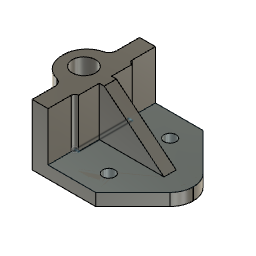
A3 v1 (Autodesk Fusion 360 design; units mm, degrees)
Autodesk Fusion 360 part; units mm, degrees
sketch "bottom" plane through (0, 0, 0) normal (0, 0, 1) x (1, 0, 0)
  line L0 (44, -44) -> (-44, -44)
  line L1 (-44, -44) -> (-44, 44)
  line L2 (-44, 44) -> (44, 44)
  line L3 (44, 44) -> (44, -44)
  line L4 (44, -44) -> (-44, 44) construction
  line L5 (-44, -44) -> (44, 44) construction
  dimension "d1" = 88
  dimension "d2" = 88
  constraint horizontal L0
  constraint perpendicular L0 L1
  constraint parallel L0 L2
  constraint parallel L1 L3
  constraint coincident L4 origin
  constraint coincident L5 origin
  measures "d1" distance of L1.end L2.end
  measures "d2" distance of L0.end L1.end
extrude "Extrude1" add sketch "bottom" along normal blind 10
sketch "Sketch2" plane through (0, 0, 10) normal (0, 0, 1) x (-1, 0, 0)
  line L0 (-44, -44) -> (44, -44)
  line L1 (44, -44) -> (44, 44)
  line L2 (44, 44) -> (-44, 44)
  line L3 (-44, 44) -> (-44, -44)
  line L4 (-44, 0) -> (-25, 0)
  circle A0 centre (-25, 0) radius 19
  constraint midpoint L3 L4.start
  constraint perpendicular L3 L4
  constraint coincident L4.end A0.centre
  constraint coincident L4.start A0
chamfer "Chamfer1" distance 36 angle 45 2 edges at (44, -44, 5) (44, 44, 5)
fillet "Fillet1" radius 19 2 edges at (44, -8, 5) (44, 8, 5)
sketch "Sketch3" plane through (0, 0, 10) normal (0, 0, 1) x (-1, 0, 0)
  line L0 (44, 44) -> (31, 44)
  line L1 (31, 44) -> (31, -44)
  line L2 (31, -44) -> (44, -44)
  line L3 (44, -44) -> (44, 44)
  constraint horizontal L0
  constraint vertical L1
  constraint horizontal L2
  constraint vertical L3
extrude "Extrude2" add sketch "Sketch3" along normal blind 40
sketch "Sketch4" plane through (0, 0, 10) normal (0, 0, 1) x (-1, 0, 0)
  line L0 (31, -44) -> (31, 44)
  line L1 (31, 44) -> (-8, 44)
  line L2 (-8, 44) -> (-38.435, 13.565)
  arc A0 (-38.435, 13.565) -> (-44, 0.1299) centre (-25, 0.1299) ccw
  line L3 (-44, 0.1299) -> (-44, -0.1299)
  arc A1 (-44, -0.1299) -> (-38.435, -13.565) centre (-25, -0.1299) ccw
  line L4 (-38.435, -13.565) -> (-8, -44)
  line L5 (-8, -44) -> (31, -44)
  line L6 (28, -22) -> (31, -22)
  line L7 (31, -22) -> (31, 22)
  line L8 (31, 22) -> (28, 22)
  line L9 (28, 22) -> (28, -22)
  dimension "d12" = 3
  constraint horizontal L6
  constraint vertical L7
  constraint horizontal L8
  constraint vertical L9
  constraint coincident L0 L7.end
  measures "d12" distance of L6.start L6.end
extrude "Extrude3" add sketch "Sketch4" along normal blind 40 contours L0 L6 L7 L8 L9
fillet "Fillet2" radius 3 1 edges at (-31, -22, 30)
fillet "Fillet3" radius 3 1 edges at (-31, 22, 30)
sketch "Sketch6" plane through (0, 0, 0) normal (0, 1, 0) x (1, 0, 0)
  line L0 (-28, -50) -> (-24, -50)
  line L1 (-24, -50) -> (-24, -10)
  line L2 (-24, -10) -> (-28, -10)
  line L3 (-28, -10) -> (-28, -50)
  dimension "d19" = 40
  constraint horizontal L0
  constraint vertical L1
  constraint horizontal L2
  constraint vertical L3
  measures "d19" distance of L0.end L1.end
extrude "Extrude4" add sketch "Sketch6" along normal mid plane 10
sketch "triangle" plane through (0, -5, 0) normal (0, -1, 0) x (1, 0, 0)
  line L0 (-28, 50) -> (-28, 10)
  line L1 (-28, 10) -> (-24, 10)
  line L2 (-24, 10) -> (-24, 50)
  line L3 (-24, 50) -> (-28, 50)
  line L4 (-24, 50) -> (-24, 10)
  line L5 (-24, 10) -> (25, 10)
  line L6 (25, 10) -> (-24, 50)
  line L7 (44, 10) -> (25, 10)
  dimension "d26" = 19
  dimension "d28" = 49
  constraint coincident L2.end L3.start
  constraint coincident L1.end L2.start
  constraint perpendicular L4 L5
  measures "d26" distance of L5.end L7.start
  measures "d28" distance of L1.end L5.end
extrude "Extrude5" add sketch "triangle" against normal blind 10 contours L2 L4 L5 L6
sketch "the back" plane through (-44, 0, 0) normal (-1, 0, 0) x (0, -1, 0)
  line L0 (-44, 0) -> (44, 0)
  line L1 (44, 0) -> (44, 50)
  line L2 (44, 50) -> (-44, 50)
  line L3 (-44, 50) -> (-44, 0)
  line L4 (-19, 50) -> (19, 50)
  line L5 (19, 50) -> (19, 0)
  line L6 (19, 0) -> (-19, 0)
  line L7 (-19, 0) -> (-19, 50)
  constraint coincident L2 L4.start
  constraint horizontal L4
  constraint vertical L5
  constraint horizontal L6
  constraint vertical L7
  constraint coincident L0 L5.end
extrude "Extrude6" add sketch "the back" along normal blind 19 contours L0 L2 L4 L5 L6 L7
fillet "Fillet4" radius 6 1 edges at (-44, -19, 25)
fillet "Fillet5" radius 6 1 edges at (-44, 19, 25)
fillet "Fillet6" radius 19 2 edges at (-63, 19, 25) (-63, -19, 25)
sketch "wall circle" plane through (0, 0, 50) normal (0, 0, 1) x (-1, 0, 0)
  arc A0 (63, 0.7307) -> (48.56, 19.1754) centre (44, 0.7307) ccw
  arc A1 (44, 25) -> (48.56, 19.1754) centre (50, 25) ccw
  line L0 (44, 25) -> (44, 44)
  line L1 (44, 44) -> (31, 44)
  line L2 (31, 44) -> (31, 25)
  arc A2 (28, 22) -> (31, 25) centre (28, 25) ccw
  line L3 (28, 22) -> (28, 5)
  line L4 (28, 5) -> (24, 5)
  line L5 (24, 5) -> (24, -5)
  line L6 (24, -5) -> (28, -5)
  line L7 (28, -5) -> (28, -22)
  arc A3 (31, -25) -> (28, -22) centre (28, -25) ccw
  line L8 (31, -25) -> (31, -44)
  line L9 (31, -44) -> (44, -44)
  line L10 (44, -44) -> (44, -25)
  arc A4 (48.56, -19.1754) -> (44, -25) centre (50, -25) ccw
  arc A5 (48.56, -19.1754) -> (63, -0.7307) centre (44, -0.7307) ccw
  line L11 (63, -0.7307) -> (63, 0.7307)
  circle A6 centre (46.3334, -0.7307) radius 9.5
  dimension "d37" = 19
  measures "d37" diameter of A6
extrude "Extrude7" cut sketch "wall circle" against normal blind 50 contours A6
sketch "bottom circles" plane through (0, 0, 10) normal (0, 0, 1) x (-1, 0, 0)
  line L0 (-25, 5) -> (28, 5)
  line L1 (28, 5) -> (28, 22)
  arc A0 (28, 22) -> (31, 25) centre (28, 25) ccw
  line L2 (31, 25) -> (31, 44)
  line L3 (31, 44) -> (-8, 44)
  line L4 (-8, 44) -> (-38.435, 13.565)
  arc A1 (-38.435, 13.565) -> (-44, 0.1299) centre (-25, 0.1299) ccw
  line L5 (-44, 0.1299) -> (-44, -0.1299)
  arc A2 (-44, -0.1299) -> (-38.435, -13.565) centre (-25, -0.1299) ccw
  line L6 (-38.435, -13.565) -> (-8, -44)
  line L7 (-8, -44) -> (31, -44)
  line L8 (31, -44) -> (31, -25)
  arc A3 (31, -25) -> (28, -22) centre (28, -25) ccw
  line L9 (28, -22) -> (28, -5)
  line L10 (28, -5) -> (-25, -5)
  line L11 (-25, -5) -> (-25, 5)
  circle A4 centre (0.1969, 25) radius 5
  circle A5 centre (0, -25) radius 5
  dimension "d43" = 10
  dimension "d44" = 10
  measures "d43" diameter of A4
  measures "d44" diameter of A5
extrude "Extrude8" cut sketch "bottom circles" against normal blind 10 contours A4 | A5
